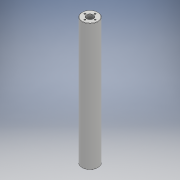
# Autodesk Inventor part: barra solida hueca
Saved by Autodesk Inventor 2018 (Build 220112000, 112)
## iProperties
Created: 2019-05-18
Part Number: barra solida hueca
Material: Generic
Document SubType Name: Modeling
Designer: JLVega003
Density: 1 g/cm^3
Appearance: Default
Author: JLVega003
Autodesk Inventor part; units mm, degrees
ref_plane "YZ Plane" through (0, 0, 0) normal (1, 0, 0) x (0, 1, 0)
ref_plane "XZ Plane" through (0, 0, 0) normal (0, 1, 0) x (-1, 0, 0)
ref_plane "XY Plane" through (0, 0, 0) normal (0, 0, 1) x (1, 0, 0)
sketch "Sketch1" plane through (0, 0, 0) normal (0, 0, 1) x (1, 0, 0)
  circle A0 centre (0, 0) radius 12.7
  circle A1 centre (0, 0) radius 5
  dimension "d0" = 25.4
  dimension "d1" = 10
  constraints: 2 centre point, 2 coincident
  measures "d0" diameter of A0
  measures "d1" diameter of A1
extrude "Extrusion1" add sketch "Sketch1" along normal mid plane 200
sketch "Sketch2" plane through (0, 0, 100) normal (0, 0, 1) x (1, 0, 0)
  line L0 (-17.78, 0) -> (17.78, 0) projected
  line L1 (0, -17.78) -> (0, 17.78) projected
  circle A0 centre (0, 0) radius 8 construction
  point P0 (0, 8)
  point P1 (8, 0)
  point P2 (0, -8)
  point P3 (-8, 0)
  dimension "d4" = 16
  constraints: 4 point on circle, 4 point on line, 1 centre point, 1 coincident
  measures "d4" diameter of A0
hole "Hole1" at (0, 8, 100) at (8, 0, 100) at (0, -8, 100) at (-8, 0, 100) direction (0, 0, -1) diameter 2.459 depth 38.1 tip angle 118 thread size "M3x0.5" class "6H" standard "ISO Metric profile"
mirror "Mirror1" about plane through (0, 0, 0) normal (0, 0, 1) of "Hole1"
chamfer "Chamfer1" distance 0.5 angle 45 4 edges at (-12.7, 0, -100) (-12.7, 0, 100) (-5, 0, -100) (-5, 0, 100)
body "Solid1"
